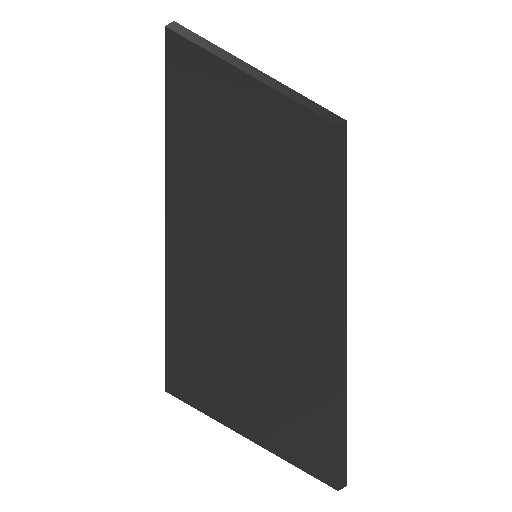
# Autodesk Inventor part: Solar Panel
Saved by Autodesk Inventor 2025 (Build 290162000, 162)
## iProperties
Created: 2025-05-01
Part Number: Solar Panel
Material: Generic
Document SubType Name: Modeling
Designer: MK92
Density: 1 g/cm^3
Appearance: Glossy - Black
Author: MK92
Autodesk Inventor part; units mm, degrees
ref_plane "YZ Plane" through (0, 0, 0) normal (1, 0, 0) x (0, 1, 0)
ref_plane "XZ Plane" through (0, 0, 0) normal (0, 1, 0) x (-1, 0, 0)
ref_plane "XY Plane" through (0, 0, 0) normal (0, 0, 1) x (1, 0, 0)
sketch "Sketch1" plane through (0, 0, 0) normal (0, 0, 1) x (1, 0, 0)
  line L0 (-11.5, 21) -> (11.5, 21)
  line L1 (11.5, 21) -> (11.5, -21)
  line L2 (11.5, -21) -> (-11.5, -21)
  line L3 (-11.5, -21) -> (-11.5, 21)
  line L4 (-11.5, 21) -> (11.5, -21) construction
  line L5 (11.5, 21) -> (-11.5, -21) construction
  point P0 (0, 0)
  dimension "d0" = 23
  dimension "d1" = 42
  constraints: 12 end point, 2 midpoint, 2 parallel, 1 horizontal, 1 perpendicular
  measures "d0" distance of L1.end L2.end
  measures "d1" distance of L0.end L1.end
extrude "Extrusion1" add sketch "Sketch1" along normal blind 1.2
body "Solid1"
